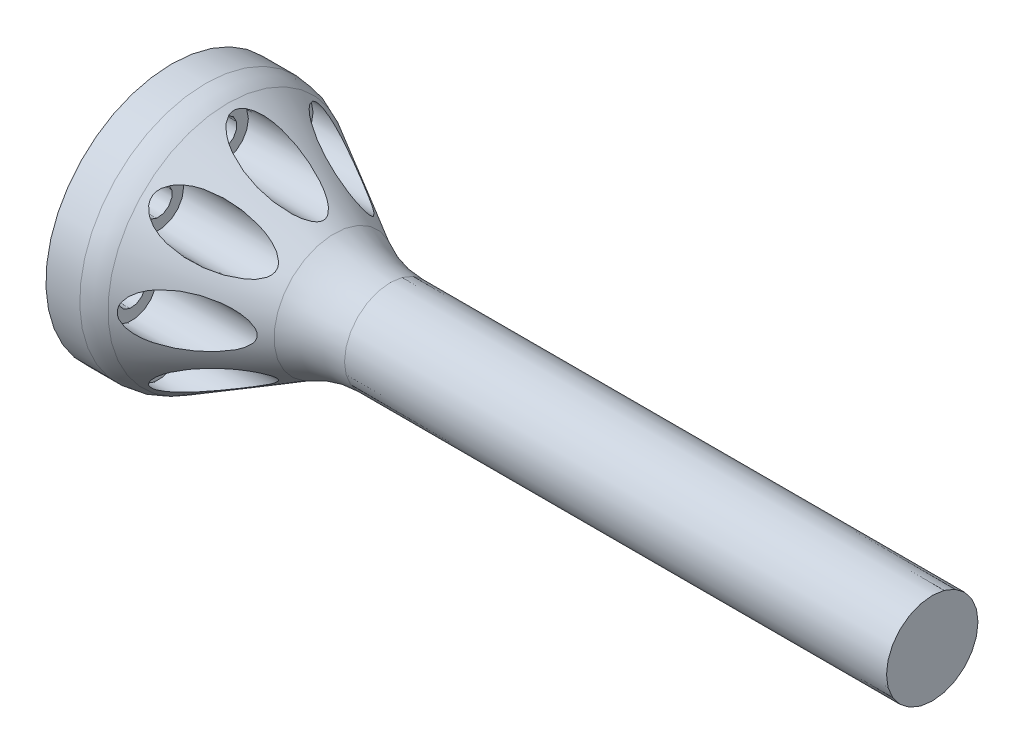
# Autodesk Inventor part: Adapter_camera
Saved by Autodesk Inventor 2017 (Build 210142000, 142)
## iProperties
Part Number: Adapter_camera
Material: Generisch
Document SubType Name: Modeling
Designer: Max
Density: 1 g/cm^3
Appearance: Vorgabe
Author: Max
Autodesk Inventor part; units mm, degrees
ref_plane "YZ Plane" through (0, 0, 0) normal (1, 0, 0) x (0, 1, 0)
sketch "Skizze1" plane through (0, 0, 0) normal (1, 0, 0) x (0, 1, 0)
  circle A0 centre (0, 0) radius 11
  dimension "d0" = 22
  constraints: 1 centre point, 1 coincident
  measures "d0" diameter of A0
extrude "Extrusion1" add sketch "Skizze1" along normal blind 4
sketch "Skizze2" plane through (4, 0, 0) normal (1, 0, 0) x (0, 0, -1)
  circle A0 centre (0, 0) radius 11 projected
ref_plane "Arbeitsebene1" through (16.5, 0, 0) normal (1, 0, 0) x (0, 0, -1)
sketch "Skizze3" plane through (16.5, 0, 0) normal (1, 0, 0) x (0, 0, -1)
  circle A0 centre (0, 0) radius 4
  dimension "d4" = 8
  constraints: 1 centre point, 1 coincident
  measures "d4" diameter of A0
loft "Erhebung1" add profiles "Skizze3" section 1 edges at (4, -11, 0)
sketch "Skizze4" plane through (16.5, 0, 0) normal (1, 0, 0) x (0, 0, -1)
  line L0 (0, 0) -> (-12.9717, 0) construction
  point P0 (-8, 0)
  point P1 (-5.6569, 5.6569)
  point P2 (0, 8)
  point P3 (5.6569, 5.6569)
  point P4 (8, 0)
  point P5 (5.6569, -5.6569)
  point P6 (0, -8)
  point P7 (-5.6569, -5.6569)
  dimension "d9" = 8
  dimension "d12" = 360
  constraints: 2 end point, 1 horizontal, 1 point on line, 9 other
  measures "d9" distance of L0.start point (-8, 0)
hole "Bohrung1" at (16.5, -5.6569, 5.6569) at (16.5, -8, 0) at (16.5, -5.6569, -5.6569) at (16.5, 0, -8) at (16.5, 5.6569, -5.6569) at (16.5, 8, 0) at (16.5, 5.6569, 5.6569) at (16.5, 0, 8) direction (-1, 0, 0) diameter 2.4 end through all counterbore diameter 4.4 counterbore depth 12 clearance for "Inbusschraube ISO 4762" size "M2" standard "ISO"
sketch "Skizze5" plane through (16.5, 0, 0) normal (1, 0, 0) x (0, 0, -1)
  circle A0 centre (0, 0) radius 4 projected
extrude "Extrusion2" add sketch "Skizze5" along normal blind 50
fillet "Rundung1" radius 10 1 edges at (16.5, -2.8284, 2.8284)
ref_plane "Arbeitsebene2" through (0, 0, -11) normal (0, 0, 1) x (1, 0, 0)
fillet "Rundung7" radius 4 1 edges at (4, -11, 0)
sketch "Skizze9" plane through (0, 0, 0) normal (-1, 0, 0) x (0, 0, 1)
  circle A0 centre (0, 0) radius 4.5
  dimension "d42" = 9
  constraints: 1 centre point, 1 coincident
  measures "d42" diameter of A0
extrude "Extrusion5" cut sketch "Skizze9" against normal blind 5
